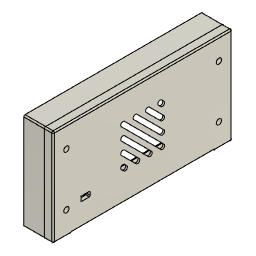
matrix (Autodesk Fusion 360 design; units mm, degrees)
Autodesk Fusion 360 part; units mm, degrees
sketch "Sketch1" plane through (0, 0, 0) normal (1, 0, 0) x (0, 1, 0) in component "Matrix"
  line L0 (96, -48) -> (-96, -48)
  line L1 (-96, -48) -> (-96, 48)
  line L2 (-96, 48) -> (96, 48)
  line L3 (96, 48) -> (96, -48)
  line L4 (96, -48) -> (-96, 48) construction
  line L5 (-96, -48) -> (96, 48) construction
  line L6 (-96, 30) -> (96, 30) construction
  line L7 (-96, -30) -> (96, -30) construction
  line L8 (-87, 48) -> (-87, -48) construction
  line L9 (87, 48) -> (87, -48) construction
  line L10 (0, 30) -> (0, -30) construction
  line L11 (-87, 0) -> (87, 0) construction
  circle A0 centre (-87, 30) radius 1.5
  circle A1 centre (-87, -30) radius 1.5
  circle A2 centre (87, -30) radius 1.5
  circle A3 centre (87, 30) radius 1.5
  line L12 (-96, 37) -> (96, 37) construction
  line L13 (-96, -37) -> (96, -37) construction
  line L14 (-12, 48) -> (-12, -48) construction
  line L15 (12, 48) -> (12, -48) construction
  circle A4 centre (12, 37) radius 1.5
  circle A5 centre (-12, -37) radius 1.5
  dimension "d3" = 192
  dimension "d4" = 96
  dimension "d5" = 9
  dimension "d6" = 18
  dimension "d7" = 3
  dimension "d9" = 12
  dimension "d10" = 11
  constraint perpendicular L0 L1
  constraint parallel L0 L2
  constraint parallel L1 L3
  constraint horizontal L0
  constraint coincident L4 origin
  constraint coincident L5 origin
  constraint coincident L1 L6.start
  constraint coincident L3 L6.end
  constraint perpendicular L3 L6
  constraint coincident L1 L7.start
  constraint coincident L3 L7.end
  constraint perpendicular L3 L7
  constraint coincident L2 L8.start
  constraint coincident L0 L8.end
  constraint perpendicular L0 L8
  constraint coincident L2 L9.start
  constraint coincident L0 L9.end
  constraint perpendicular L0 L9
  constraint perpendicular L6 L10
  constraint perpendicular L10 L11
  constraint symmetric L6 L7 L11
  constraint midpoint origin L11
  constraint midpoint origin L10
  constraint midpoint L6 L10.start
  constraint coincident L8 L11.start
  constraint coincident L8 A0.centre
  constraint coincident L6 A0.centre
  constraint coincident L7 A1.centre
  constraint coincident L8 A1.centre
  constraint coincident L9 A2.centre
  constraint coincident L7 A2.centre
  constraint coincident L6 A3.centre
  constraint coincident L9 A3.centre
  constraint equal A2 A3
  constraint equal A0 A3
  constraint equal A0 A1
  constraint coincident L1 L12.start
  constraint coincident L3 L12.end
  constraint perpendicular L3 L12
  constraint coincident L1 L13.start
  constraint coincident L3 L13.end
  constraint perpendicular L3 L13
  constraint coincident L2 L14.start
  constraint coincident L0 L14.end
  constraint perpendicular L0 L14
  constraint coincident L2 L15.start
  constraint coincident L0 L15.end
  constraint perpendicular L0 L15
  constraint symmetric L11 L12 L13
  constraint coincident L12 A4.centre
  constraint coincident L15 A4.centre
  constraint coincident L13 A5.centre
  constraint coincident L14 A5.centre
  constraint equal A4 A5
  constraint equal A0 A5
  measures "d3" distance of L1.end L2.end
  measures "d4" distance of L0.start L2.end
  measures "d5" distance of L1 L8
  measures "d6" distance of L0 L7
  measures "d7" diameter of A0
  measures "d9" distance of L10 L15
  measures "d10" distance of L2 L12
sketch "Sketch3" plane through (0, 0, 0) normal (1, 0, 0) x (0, 1, 0) in component "Matrix"
  line L0 (96, -48) -> (-96, -48)
  line L1 (-96, -48) -> (-96, 48)
  line L2 (96, 48) -> (96, -48)
  line L3 (-96, 48) -> (96, 48)
  circle A0 centre (-87, 30) radius 1.5
  circle A1 centre (-87, -30) radius 1.5
  circle A2 centre (87, -30) radius 1.5
  circle A3 centre (87, 30) radius 1.5
  line L4 (0, 30) -> (0, -30) construction
  line L5 (-87, 0) -> (87, 0) construction
  line L6 (82.25, -35.25) -> (-82.25, -35.25)
  line L7 (-82.25, -35.25) -> (-82.25, 35.25)
  line L8 (-82.25, 35.25) -> (82.25, 35.25)
  line L9 (82.25, 35.25) -> (82.25, -35.25)
  line L10 (82.25, -35.25) -> (-82.25, 35.25) construction
  line L11 (-82.25, -35.25) -> (82.25, 35.25) construction
  circle A4 centre (12, 37) radius 1.5
  circle A5 centre (-12, -37) radius 1.5
  circle A6 centre (-12, -37) radius 4
  circle A7 centre (12, 37) radius 4
  point P0 (-87, -30)
  dimension "d15" = 12.75
  dimension "d16" = 13.75
  dimension "d18" = 8
  constraint perpendicular L6 L7
  constraint parallel L6 L8
  constraint parallel L7 L9
  constraint horizontal L6
  constraint coincident L10 origin
  constraint coincident L11 origin
  constraint concentric A5 A6
  constraint concentric A4 A7
  constraint equal A6 A7
  measures "d15" distance of L3 L8
  measures "d16" distance of L2 L9
  measures "d18" diameter of A6
extrude "Extrude3" add sketch "Sketch3" along normal mid plane 15 contours L0 L1 L2 L3 | A0 | A1 | A2 | A3 | L6 L7 L8 L9 A6 A7 | L6 A6 | L6 A6 | L8 A7 | L8 A7 | A4 | A5 makes body 1 in component "Matrix"
extrude "Extrude4" cut sketch "Sketch3" against normal blind 13 from surface at 7.5 contours L6 L7 L8 L9 A6 A7 bodies 1 in component "Matrix"
extrude "Extrude5" cut sketch "Sketch3" against normal blind 5 from surface at 7.5 contours A0 | A1 | A2 | A3 | A4 | A5 bodies 1 in component "Matrix"
sketch "Sketch1 (2)" plane through (7.5, 0, 0) normal (1, 0, 0) x (0, 1, 0) in component "Fit Test"
  circle A0 centre (87, -30) radius 1.5 construction
  circle A1 centre (87, 30) radius 1.5 construction
  line L0 (96, -48) -> (96, 48) construction
  circle A2 centre (87, 30) radius 1.875
  circle A3 centre (87, -30) radius 1.875
  line L1 (96.5, -48) -> (96.5, 48)
  circle A4 centre (87, 30) radius 5
  circle A5 centre (87, -30) radius 5
  line L2 (87, 35) -> (98.5, 35)
  line L3 (98.5, 35) -> (98.5, -35)
  line L4 (98.5, -35) -> (87, -35)
  line L5 (87, 30) -> (87, -30)
  dimension "d51" = 3.75
  dimension "d52" = 0.5
  dimension "d53" = 10
  dimension "d54" = 2
  constraint concentric A1 A2
  constraint concentric A0 A3
  constraint equal A2 A3
  constraint concentric A1 A4
  constraint concentric A0 A5
  constraint equal A4 A5
  constraint coincident A4 L2.start
  constraint perpendicular L0 L2
  constraint perpendicular L2 L3
  constraint coincident A5 L4.end
  constraint tangent A5 L4
  constraint horizontal L4
  constraint tangent A4 L2
  constraint coincident A1.centre A2.centre
  constraint coincident A0.centre A3.centre
  measures "d51" diameter of A2
  measures "d53" diameter of A4
  measures "d54" distance of L1 L3
extrude "Extrude1" add sketch "Sketch1 (2)" along normal blind 2 separate body makes body 2 in component "Fit Test"
extrude "Extrude2" add sketch "Sketch1 (2)" against normal blind 3 contours L1 L2 L3 L4 bodies 2 in component "Fit Test"
ref_plane "WorkPlane1" through (-8, 0, 0) normal (-1, 0, 0) x (0, 0, 1) in component "Perspex"
sketch "Sketch1 (3)" plane through (-8, 0, 0) normal (-1, 0, 0) x (0, 1, 0) in component "Perspex"
  line L0 (-99, 51) -> (99, 51)
  line L1 (99, 51) -> (99, -51)
  line L2 (99, -51) -> (-99, -51)
  line L3 (-99, -51) -> (-99, 51)
  line L4 (-99, 51) -> (99, -51) construction
  line L5 (99, 51) -> (-99, -51) construction
  dimension "d28" = 198
  dimension "d29" = 102
  constraint perpendicular L0 L1
  constraint parallel L0 L2
  constraint parallel L1 L3
  constraint horizontal L0
  constraint coincident L4 origin
  constraint coincident L5 origin
  measures "d28" distance of L1.end L2.end
  measures "d29" distance of L0 L2
extrude "Extrude1'" add sketch "Sketch1 (3)" along normal blind 3 separate body makes body 3 in component "Perspex"
sketch "Sketch1 (4)" plane through (-8, 0, 0) normal (1, 0, 0) x (0, 1, 0) in component "Case"
  line L0 (99, 51) -> (-99, 51) construction
  line L1 (-99, 51) -> (-99, -51) construction
  line L2 (-99, -51) -> (99, -51) construction
  line L3 (99, -51) -> (99, 51) construction
  line L4 (96, 48) -> (-96, 48) construction
  line L5 (-96, 48) -> (-96, -48) construction
  line L6 (-96, -48) -> (96, -48) construction
  line L7 (96, -48) -> (96, 48) construction
  line L8 (-96.2, -48.2) -> (96.2, -48.2)
  line L9 (96.2, -48.2) -> (96.2, 48.2)
  line L10 (96.2, 48.2) -> (-96.2, 48.2)
  line L11 (-96.2, 48.2) -> (-96.2, -48.2)
  line L12 (-99.2, -51.2) -> (99.2, -51.2)
  line L13 (99.2, -51.2) -> (99.2, 51.2)
  line L14 (99.2, 51.2) -> (-99.2, 51.2)
  line L15 (-99.2, 51.2) -> (-99.2, -51.2)
  line L16 (102.2, -54.2) -> (-102.2, -54.2)
  line L17 (-102.2, -54.2) -> (-102.2, 54.2)
  line L18 (-102.2, 54.2) -> (102.2, 54.2)
  line L19 (102.2, 54.2) -> (102.2, -54.2)
  line L20 (102.2, -54.2) -> (-102.2, 54.2) construction
  line L21 (-102.2, -54.2) -> (102.2, 54.2) construction
  dimension "d32" = 0.2
  dimension "d33" = 0.2
  dimension "d34" = 3
  dimension "d35" = 3
  constraint perpendicular L16 L17
  constraint parallel L16 L18
  constraint parallel L17 L19
  constraint horizontal L16
  constraint coincident L20 origin
  constraint coincident L21 origin
  measures "d34" distance of L14 L18
  measures "d35" distance of L13 L19
extrude "Extrude1''" add sketch "Sketch1 (4)" against normal up to surface (4 mm away) separate body contours L16 L17 L18 L19 makes body 4 in component "Case"
extrude "Extrude2'" add sketch "Sketch1 (4)" along normal up to surface (15.5 mm away) contours L12 L13 L14 L15 | L16 L17 L18 L19 bodies 4 in component "Case"
sketch "Sketch2" plane through (7.5, 0, 0) normal (1, 0, 0) x (0, 1, 0) in component "Case"
  circle A0 centre (-87, 30) radius 1.5 construction
  circle A1 centre (-87, -30) radius 1.5 construction
  circle A2 centre (87, -30) radius 1.5 construction
  circle A3 centre (87, 30) radius 1.5 construction
  line L0 (96.2, -48.2) -> (-96.2, -48.2)
  line L1 (-96.2, -48.2) -> (-96.2, 48.2)
  line L2 (-96.2, 48.2) -> (96.2, 48.2)
  line L3 (96.2, 48.2) -> (96.2, -48.2)
  line L4 (102.2, -54.2) -> (102.2, 54.2)
  line L5 (102.2, 54.2) -> (-102.2, 54.2)
  line L6 (-102.2, 54.2) -> (-102.2, -54.2)
  line L7 (-102.2, -54.2) -> (102.2, -54.2)
  line L8 (-87, 34.25) -> (-96.2, 34.25)
  line L9 (-87, 25.75) -> (-96.2, 25.75)
  line L10 (-87, -25.75) -> (-96.2, -25.75)
  line L11 (-87, -34.25) -> (-96.2, -34.25)
  line L12 (87, 34.25) -> (96.2, 34.25)
  line L13 (87, 25.75) -> (96.2, 25.75)
  line L14 (87, -25.75) -> (96.2, -25.75)
  line L15 (87, -34.25) -> (96.2, -34.25)
  arc A4 (-87, 25.75) -> (-87, 34.25) centre (-87, 30) ccw
  arc A5 (-87, -34.25) -> (-87, -25.75) centre (-87, -30) ccw
  arc A6 (87, -25.75) -> (87, -34.25) centre (87, -30) ccw
  arc A7 (87, 34.25) -> (87, 25.75) centre (87, 30) ccw
  circle A8 centre (-87, 30) radius 1.75
  circle A9 centre (-87, -30) radius 1.75
  circle A10 centre (87, -30) radius 1.75
  circle A11 centre (87, 30) radius 1.75
  dimension "d42" = 3.5
  dimension "d289" = 2.5
  constraint concentric A0 A4
  constraint concentric A1 A5
  constraint concentric A2 A6
  constraint concentric A3 A7
  constraint equal A6 A7
  constraint equal A4 A7
  constraint equal A4 A5
  constraint coincident L1 L8.end
  constraint tangent L8 A4
  constraint coincident L1 L9.end
  constraint tangent L9 A4
  constraint coincident L1 L10.end
  constraint tangent L10 A5
  constraint coincident L1 L11.end
  constraint tangent L11 A5
  constraint coincident L3 L12.end
  constraint tangent L12 A7
  constraint coincident L3 L13.end
  constraint tangent L13 A7
  constraint coincident L3 L14.end
  constraint tangent L14 A6
  constraint coincident L3 L15.end
  constraint tangent L15 A6
  constraint parallel L13 L15
  constraint perpendicular L3 L12
  constraint perpendicular L3 L13
  constraint perpendicular L3 L14
  constraint perpendicular L1 L8
  constraint perpendicular L1 L9
  constraint perpendicular L1 L10
  constraint perpendicular L1 L11
  constraint concentric A0 A8
  constraint concentric A1 A9
  constraint concentric A2 A10
  constraint concentric A7 A11
  constraint equal A8 A9
  constraint equal A8 A11
  constraint equal A10 A11
  measures "d42" diameter of A8
  measures "d289" distance of A4 A8
extrude "Extrude3'" add sketch "Sketch2" along normal blind 4 contours L3 L14 L15 A6 | L1 L10 L11 A5 | L3 L12 L13 A7 | L1 L8 L9 A4 | L4 L5 L6 L7 bodies 4 in component "Case"
ref_plane "WorkPlane1" through (7.5, 0, 0) normal (1, 0, 0) x (0, 0, -1) in component "Case"
sketch "Sketch4" plane through (7.5, 0, 0) normal (1, 0, 0) x (0, 1, 0) in component "Case"
  line L0 (-96, 48) -> (-96, -48) construction
  line L1 (96.2, -48.2) -> (-96.2, -48.2)
  circle A0 centre (-18.5, -29) radius 1.75
  line L2 (-96.2, 48.2) -> (96.2, 48.2)
  line L3 (-21.7368, -28.7072) -> (-23.5, -48.2)
  line L4 (-15.2632, -28.7072) -> (-13.5, -48.2)
  arc A1 (-15.2632, -28.7072) -> (-21.7368, -28.7072) centre (-18.5, -29) ccw
  line L5 (30.5, 29) -> (-18.5, -29) construction
  line L6 (6, 0) -> (6, 48.2) construction
  line L7 (-18.5, -29) -> (-18.5, -48.2) construction
  line L8 (6, 0) -> (-75.1165, 0) construction
  dimension "d69" = 49
  dimension "d73" = 58
  dimension "d190" = 3.5
  dimension "d194" = 10
  dimension "d291" = 1.5
  dimension "d322" = 6
  constraint concentric A0 A1
  constraint coincident L1 L3.end
  constraint tangent L3 A1
  constraint coincident L1 L4.end
  constraint tangent L4 A1
  constraint vertical L6
  constraint coincident A0.centre A1.centre
  constraint coincident L1 L7.end
  constraint perpendicular L1 L7
  constraint symmetric L3 L4 L7
  constraint horizontal L8
  constraint coincident L5 L6.start
  constraint coincident origin L8
  constraint coincident L2 L6.end
  constraint midpoint L5 L6.start
  measures "d69" horizontal distance of A0.centre L5.start
  measures "d73" vertical distance of A0.centre L5.start
  measures "d190" diameter of A0
  measures "d194" distance of L3.end L4.end
  measures "d291" distance of A0 A1
  measures "d322" distance of origin L6.start
extrude "Extrude5'" add sketch "Sketch4" along normal up to surface (4 mm away) bodies 4 in component "Case"
mirror "Mirror3" about plane through (0, 0, 0) normal (0, 0, 1) of "Extrude5'" in component "Case"
ref_plane "WorkPlane2" through (7.5, 6, 0) normal (0, -1, 0) x (1, 0, 0) in component "Case"
mirror "Mirror4" about plane through (7.5, 6, 0) normal (0, -1, 0) of "Extrude5'", "Mirror3" in component "Case"
sketch "Sketch7" plane through (11.5, 0, 0) normal (1, 0, 0) x (0, 1, 0) in component "Case"
  line L0 (-96.2, 48.2) -> (-23.5, 48.2)
  line L1 (96.2, 48.2) -> (96.2, 34.25)
  line L2 (96.2, 34.25) -> (87, 34.25)
  arc A0 (87, 34.25) -> (87, 25.75) centre (87, 30) ccw
  line L3 (87, 25.75) -> (96.2, 25.75)
  line L4 (96.2, -25.75) -> (87, -25.75)
  arc A1 (87, -25.75) -> (87, -34.25) centre (87, -30) ccw
  line L5 (87, -34.25) -> (96.2, -34.25)
  line L6 (96.2, -48.2) -> (35.5, -48.2)
  line L7 (-96.2, 34.25) -> (-96.2, 48.2)
  line L8 (-96.2, -34.25) -> (-87, -34.25)
  arc A2 (-87, -34.25) -> (-87, -25.75) centre (-87, -30) ccw
  line L9 (-87, -25.75) -> (-96.2, -25.75)
  line L10 (-96.2, 25.75) -> (-87, 25.75)
  arc A3 (-87, 25.75) -> (-87, 34.25) centre (-87, 30) ccw
  line L11 (-87, 34.25) -> (-96.2, 34.25)
  circle A4 centre (-87, -30) radius 1.75
  circle A5 centre (87, 30) radius 1.75
  circle A6 centre (87, -30) radius 1.75
  circle A7 centre (-87, 30) radius 1.75
  line L12 (-102.2, -54.2) -> (102.2, -54.2)
  line L13 (102.2, -54.2) -> (102.2, 54.2)
  line L14 (102.2, 54.2) -> (-102.2, 54.2)
  line L15 (-102.2, 54.2) -> (-102.2, -54.2)
  line L16 (17.694, -48.2) -> (35.5, -48.2)
  line L17 (35.5, -48.2) -> (35.5, -17.1281)
  line L18 (35.5, -17.1281) -> (17.694, -17.1281)
  line L19 (17.694, -17.1281) -> (17.694, -48.2)
  line L20 (-29.5, 48.2) -> (-8.6042, 48.2)
  line L21 (-8.6042, 48.2) -> (-8.6042, 21.8764)
  line L22 (-8.6042, 21.8764) -> (-29.5, 21.8764)
  line L23 (-29.5, 21.8764) -> (-29.5, 48.2)
  circle A8 centre (30.5, 29) radius 1.75
  circle A9 centre (-18.5, 29) radius 1.75
  circle A10 centre (-18.5, -29) radius 1.75
  line L24 (-23.5, 48.2) -> (-21.7368, 28.7072)
  arc A11 (-21.7368, 28.7072) -> (-15.2632, 28.7072) centre (-18.5, 29) ccw
  line L25 (-15.2632, 28.7072) -> (-13.5, 48.2)
  line L26 (-13.5, 48.2) -> (25.5, 48.2)
  line L27 (25.5, 48.2) -> (27.2632, 28.7072)
  arc A12 (27.2632, 28.7072) -> (33.7368, 28.7072) centre (30.5, 29) ccw
  line L28 (33.7368, 28.7072) -> (35.5, 48.2)
  line L29 (96.2, 25.75) -> (96.2, -25.75)
  line L30 (96.2, -34.25) -> (96.2, -48.2)
  line L31 (-13.5, -48.2) -> (-15.2632, -28.7072)
  arc A13 (-15.2632, -28.7072) -> (-21.7368, -28.7072) centre (-18.5, -29) ccw
  line L32 (-21.7368, -28.7072) -> (-23.5, -48.2)
  line L33 (-23.5, -48.2) -> (-96.2, -48.2)
  line L34 (-96.2, -25.75) -> (-96.2, 25.75)
  circle A14 centre (30.5, -29) radius 1.75
  line L35 (35.5, 48.2) -> (96.2, 48.2)
  line L36 (35.5, -48.2) -> (33.7368, -28.7072)
  arc A15 (33.7368, -28.7072) -> (27.2632, -28.7072) centre (30.5, -29) ccw
  line L37 (27.2632, -28.7072) -> (25.5, -48.2)
  line L38 (25.5, -48.2) -> (-13.5, -48.2)
  line L39 (-96.2, -48.2) -> (-96.2, -34.25)
  constraint horizontal L16
  constraint vertical L17
  constraint horizontal L18
  constraint vertical L19
  constraint coincident L6.end L17
  constraint horizontal L20
  constraint vertical L21
  constraint horizontal L22
  constraint vertical L23
extrude "Extrude13" cut sketch "Sketch7" against normal blind 13 contours L0 L20 L21 L22 L23 L24 A11 L25 L26 | L20 L24 A11 L25 | L16 L17 L18 L19 L36 A15 L37 L38 | L16 L36 A15 L37 | A9 | A14 bodies 4 in component "Case"
sketch "Sketch11" plane through (0, 0, -54.2) normal (0, 0, -1) x (1, 0, 0) in component "Case"
  line L0 (-12, 102.2) -> (-12, -102.2)
  line L1 (-12, -102.2) -> (11.5, -102.2)
  line L2 (11.5, -102.2) -> (11.5, 102.2)
  line L3 (11.5, 102.2) -> (-12, 102.2)
  line L4 (-12, 82.2) -> (11.5, 82.2)
  dimension "d295" = 20
  constraint coincident L0 L4.start
  constraint coincident L2 L4.end
  constraint perpendicular L2 L4
  measures "d295" distance of L3 L4
extrude "Extrude16" add sketch "Sketch11" along normal blind 2 contours L0 L2 L3 L4 bodies 4 in component "Case"
mirror "Mirror5" about plane through (0, 0, 0) normal (0, 1, 0) of "Extrude16" in component "Case"
fillet "Fillet7" radius 1 2 edges at (-0.25, -82.2, -54.2) (-0.25, 82.2, -54.2) on bodies 4 in component "Case"
sketch "Sketch1 (5)" plane through (11.5, 0, 0) normal (1, 0, 0) x (0, 1, 0) in component "Back"
  line L0 (-81.2, -54.2) -> (81.2, -54.2)
  arc A0 (82.2, -55.2) -> (81.2, -54.2) centre (81.2, -55.2) ccw
  line L1 (82.2, -55.2) -> (82.2, -56.2)
  line L2 (82.2, -56.2) -> (102.2, -56.2)
  line L3 (102.2, -56.2) -> (102.2, 54.2)
  line L4 (102.2, 54.2) -> (-102.2, 54.2)
  line L5 (-102.2, 54.2) -> (-102.2, -56.2)
  line L6 (-102.2, -56.2) -> (-82.2, -56.2)
  line L7 (-82.2, -56.2) -> (-82.2, -55.2)
  arc A1 (-81.2, -54.2) -> (-82.2, -55.2) centre (-81.2, -55.2) ccw
  circle A2 centre (87, -30) radius 1.75
  circle A3 centre (87, 30) radius 1.75
  circle A4 centre (-87, 30) radius 1.75
  line L8 (96.2, -48.2) -> (-13.5, -48.2)
  line L9 (-96.2, -48.2) -> (-96.2, -34.25)
  line L10 (-96.2, 25.75) -> (-87, 25.75)
  arc A5 (-87, 25.75) -> (-87, 34.25) centre (-87, 30) ccw
  line L11 (-87, 34.25) -> (-96.2, 34.25)
  line L12 (-96.2, 48.2) -> (25.5, 48.2)
  line L13 (96.2, 48.2) -> (96.2, 34.25)
  line L14 (96.2, 34.25) -> (87, 34.25)
  arc A6 (87, 34.25) -> (87, 25.75) centre (87, 30) ccw
  line L15 (87, 25.75) -> (96.2, 25.75)
  line L16 (96.2, -25.75) -> (87, -25.75)
  arc A7 (87, -25.75) -> (87, -34.25) centre (87, -30) ccw
  line L17 (87, -34.25) -> (96.2, -34.25)
  line L18 (25.5, 48.2) -> (35.5, 48.2)
  line L19 (-29.5, -48.2) -> (-13.5, -48.2)
  line L20 (-13.5, -48.2) -> (-15.2632, -28.7072)
  arc A8 (-15.2632, -28.7072) -> (-21.7368, -28.7072) centre (-18.5, -29) ccw
  line L21 (-21.7368, -28.7072) -> (-23.5, -48.2)
  line L22 (-23.5, -48.2) -> (-96.2, -48.2)
  line L23 (-96.2, -34.25) -> (-87, -34.25)
  arc A9 (-87, -34.25) -> (-87, -25.75) centre (-87, -30) ccw
  line L24 (-87, -25.75) -> (-96.2, -25.75)
  line L25 (-96.2, -25.75) -> (-96.2, 25.75)
  line L26 (-96.2, 34.25) -> (-96.2, 48.2)
  line L27 (25.5, 48.2) -> (27.2632, 28.7072)
  arc A10 (27.2632, 28.7072) -> (33.7368, 28.7072) centre (30.5, 29) ccw
  line L28 (33.7368, 28.7072) -> (35.5, 48.2)
  line L29 (35.5, 48.2) -> (96.2, 48.2)
  line L30 (96.2, 25.75) -> (96.2, -25.75)
  line L31 (96.2, -34.25) -> (96.2, -48.2)
  circle A11 centre (30.5, 29) radius 1.75
  circle A12 centre (-18.5, -29) radius 1.75
  circle A13 centre (-87, -30) radius 1.75
  constraint coincident L12.end L18.start
  constraint coincident L8.end L19.end
  constraint coincident L18.end L28.end
extrude "Extrude1'''" add sketch "Sketch1 (5)" along normal blind 8 separate body contours L0 A0 L1 L2 L3 L4 L5 L6 L7 A1 makes body 5 in component "Back"
sketch "Sketch13" plane through (19.5, 0, 0) normal (1, 0, 0) x (0, 1, 0) in component "Back"
  circle A0 centre (87, -30) radius 1.75
  line L0 (96.2, -48.2) -> (-96.2, -48.2) construction
  line L1 (-96.2, -48.2) -> (-96.2, -34.25) construction
  line L2 (-96.2, 25.75) -> (-87, 25.75) construction
  arc A1 (-87, 25.75) -> (-87, 34.25) centre (-87, 30) ccw construction
  line L3 (-87, 34.25) -> (-96.2, 34.25) construction
  line L4 (-96.2, 48.2) -> (96.2, 48.2) construction
  line L5 (96.2, 48.2) -> (96.2, 34.25) construction
  line L6 (96.2, 34.25) -> (87, 34.25) construction
  arc A2 (87, 34.25) -> (87, 25.75) centre (87, 30) ccw construction
  line L7 (87, 25.75) -> (96.2, 25.75) construction
  line L8 (96.2, -25.75) -> (87, -25.75) construction
  arc A3 (87, -25.75) -> (87, -34.25) centre (87, -30) ccw construction
  line L9 (87, -34.25) -> (96.2, -34.25) construction
  circle A4 centre (-87, 30) radius 1.75
  circle A5 centre (87, 30) radius 1.75
  line L10 (82.2, -55.2) -> (82.2, -56.2)
  line L11 (82.2, -56.2) -> (102.2, -56.2)
  line L12 (102.2, -56.2) -> (102.2, 54.2)
  line L13 (102.2, 54.2) -> (-102.2, 54.2)
  line L14 (-102.2, 54.2) -> (-102.2, -56.2)
  line L15 (-102.2, -56.2) -> (-82.2, -56.2)
  line L16 (-82.2, -56.2) -> (-82.2, -55.2)
  arc A6 (-81.2, -54.2) -> (-82.2, -55.2) centre (-81.2, -55.2) ccw
  line L17 (-81.2, -54.2) -> (81.2, -54.2)
  arc A7 (82.2, -55.2) -> (81.2, -54.2) centre (81.2, -55.2) ccw
  line L18 (-96.2, -34.25) -> (-87, -34.25)
  arc A8 (-87, -34.25) -> (-87, -25.75) centre (-87, -30) ccw
  line L19 (-87, -25.75) -> (-96.2, -25.75)
  line L20 (-96.2, -25.75) -> (-96.2, 25.75)
  line L21 (-96.2, 34.25) -> (-96.2, 48.2)
  line L22 (96.2, 25.75) -> (96.2, -25.75)
  line L23 (96.2, -34.25) -> (96.2, -48.2)
  circle A9 centre (-87, -30) radius 1.75
  line L24 (96.2, 48.2) -> (106.2, 48.2)
  constraint coincident L4.end L5.start
extrude "Extrude12" add sketch "Sketch13" along normal blind 2 bodies 5 in component "Back"
sketch "Sketch15" plane through (21.5, 0, 0) normal (1, 0, 0) x (0, 1, 0) in component "Back"
  circle A0 centre (87, -30) radius 1.75
  circle A1 centre (-87, 30) radius 1.75
  circle A2 centre (87, 30) radius 1.75
  line L0 (82.2, -56.2) -> (102.2, -56.2)
  line L1 (102.2, -56.2) -> (102.2, 54.2)
  line L2 (102.2, 54.2) -> (-102.2, 54.2)
  line L3 (-102.2, 54.2) -> (-102.2, -56.2)
  line L4 (-102.2, -56.2) -> (-82.2, -56.2)
  line L5 (-82.2, -56.2) -> (-82.2, -55.2)
  arc A3 (-81.2, -54.2) -> (-82.2, -55.2) centre (-81.2, -55.2) ccw
  line L6 (-81.2, -54.2) -> (81.2, -54.2)
  arc A4 (82.2, -55.2) -> (81.2, -54.2) centre (81.2, -55.2) ccw
  line L7 (82.2, -55.2) -> (82.2, -56.2)
  circle A5 centre (-87, 30) radius 1.75
  circle A6 centre (87, 30) radius 1.75
  circle A7 centre (87, -30) radius 1.75
  circle A8 centre (-87, 30) radius 3
  circle A9 centre (-87, -30) radius 3
  circle A10 centre (87, -30) radius 3
  circle A11 centre (87, 30) radius 3
  circle A12 centre (-87, -30) radius 1.75
  circle A13 centre (-87, -30) radius 1.75
  dimension "d316" = 6
  constraint coincident A1.centre A5.centre
  constraint concentric A7 A10
  constraint concentric A2 A11
  constraint equal A8 A9
  constraint equal A9 A10
  constraint equal A10 A11
  constraint coincident A9.centre A12.centre
  measures "d316" diameter of A8
extrude "Extrude14" cut sketch "Sketch15" against normal up to surface (8 mm away) contours A8 | A9 | A10 | A11 bodies 5 in component "Back"
sketch "Sketch6" plane through (19.5, 0, 0) normal (-1, 0, 0) x (0, -1, 0) in component "Back"
  line L0 (70.25, -30.25) -> (59.85, -30.25)
  line L1 (59.85, -30.25) -> (59.85, -24.85)
  line L2 (59.85, -24.85) -> (70.25, -24.85)
  line L3 (70.25, -24.85) -> (70.25, -30.25)
  line L4 (70.25, -30.25) -> (59.85, -24.85) construction
  line L5 (59.85, -30.25) -> (70.25, -24.85) construction
  line L6 (-96.2, -48.2) -> (96.2, -48.2)
  line L7 (96.2, -48.2) -> (96.2, -34.25)
  line L8 (96.2, 25.75) -> (87, 25.75)
  arc A0 (87, 34.25) -> (87, 25.75) centre (87, 30) ccw
  line L9 (87, 34.25) -> (96.2, 34.25)
  line L10 (96.2, 48.2) -> (-96.2, 48.2)
  line L11 (-96.2, 48.2) -> (-96.2, 34.25)
  line L12 (-96.2, 34.25) -> (-87, 34.25)
  arc A1 (-87, 25.75) -> (-87, 34.25) centre (-87, 30) ccw
  line L13 (-87, 25.75) -> (-96.2, 25.75)
  line L14 (-96.2, -25.75) -> (-87, -25.75)
  arc A2 (-87, -34.25) -> (-87, -25.75) centre (-87, -30) ccw
  line L15 (-87, -34.25) -> (-96.2, -34.25)
  line L16 (-82.25, -35.25) -> (8.4031, -35.25)
  line L17 (-82.25, 35.25) -> (-82.25, -35.25)
  line L18 (-96.2, -34.25) -> (-96.2, -48.2)
  line L19 (96.2, -34.25) -> (87, -34.25)
  arc A3 (87, -25.75) -> (87, -34.25) centre (87, -30) ccw
  line L20 (87, -25.75) -> (96.2, -25.75)
  line L21 (96.2, -25.75) -> (96.2, 25.75)
  line L22 (96.2, 34.25) -> (96.2, 48.2)
  line L23 (-96.2, 25.75) -> (-96.2, -25.75)
  line L24 (82.25, -35.25) -> (82.25, 35.25)
  point P0 (65.05, -27.55)
  dimension "d150" = 10.4
  dimension "d151" = 5.4
  dimension "d303" = 5
  dimension "d326" = 12
  constraint perpendicular L0 L1
  constraint parallel L0 L2
  constraint parallel L1 L3
  constraint horizontal L0
  constraint coincident L4 P0
  constraint coincident L5 P0
  measures "d150" distance of L1.end L2.end
  measures "d151" distance of L0.start L2.end
  measures "d303" distance of L0 L16
  measures "d326" distance of L3 L24
extrude "Extrude7" cut sketch "Sketch6" against normal blind 13 contours L0 L1 L2 L3 bodies 5 in component "Back"
chamfer "Chamfer1" distance 1 angle 45 2 edges at (20.5, -59.85, -24.85) (20.5, -59.85, -30.25) on bodies 5 in component "Back"
sketch "Sketch16" plane through (19.5, 0, 0) normal (-1, 0, 0) x (0, -1, 0) in component "Back"
  line L0 (59.85, -29.25) -> (59.85, -25.85)
  line L1 (59.85, -25.85) -> (60.85, -24.85)
  line L2 (60.85, -24.85) -> (70.25, -24.85)
  line L3 (70.25, -24.85) -> (70.25, -30.25)
  line L4 (70.25, -30.25) -> (60.85, -30.25)
  line L5 (60.85, -30.25) -> (59.85, -29.25)
  line L6 (-96.2, -34.25) -> (-96.2, -48.2)
  line L7 (-96.2, -48.2) -> (96.2, -48.2)
  line L8 (96.2, -48.2) -> (96.2, -34.25)
  line L9 (96.2, -34.25) -> (87, -34.25)
  arc A0 (87, -25.75) -> (87, -34.25) centre (87, -30) ccw
  line L10 (87, -25.75) -> (96.2, -25.75)
  line L11 (96.2, -25.75) -> (96.2, 25.75)
  line L12 (96.2, 25.75) -> (87, 25.75)
  arc A1 (87, 34.25) -> (87, 25.75) centre (87, 30) ccw
  line L13 (87, 34.25) -> (96.2, 34.25)
  line L14 (96.2, 34.25) -> (96.2, 48.2)
  line L15 (96.2, 48.2) -> (-96.2, 48.2)
  line L16 (-96.2, 48.2) -> (-96.2, 34.25)
  line L17 (-96.2, 34.25) -> (-87, 34.25)
  arc A2 (-87, 25.75) -> (-87, 34.25) centre (-87, 30) ccw
  line L18 (-87, 25.75) -> (-96.2, 25.75)
  line L19 (-96.2, 25.75) -> (-96.2, -25.75)
  line L20 (-96.2, -25.75) -> (-87, -25.75)
  arc A3 (-87, -34.25) -> (-87, -25.75) centre (-87, -30) ccw
  line L21 (-87, -34.25) -> (-96.2, -34.25)
  line L22 (72.25, -32.25) -> (60.0216, -32.25)
  line L23 (60.0216, -32.25) -> (57.85, -30.0784)
  line L24 (57.85, -30.0784) -> (57.85, -25.0216)
  line L25 (57.85, -25.0216) -> (60.0216, -22.85)
  line L26 (60.0216, -22.85) -> (72.25, -22.85)
  line L27 (72.25, -22.85) -> (72.25, -32.25)
  dimension "d323" = -2
extrude "Extrude15" add sketch "Sketch16" along normal blind 2 contours L22 L23 L24 L25 L26 L27 bodies 5 in component "Back"
sketch "Sketch14" plane through (19.5, 0, 0) normal (-1, 0, 0) x (0, -1, 0) in component "Back"
  line L0 (-96.2, -48.2) -> (96.2, -48.2)
  line L1 (96.2, -48.2) -> (96.2, -34.25)
  line L2 (96.2, 25.75) -> (87, 25.75)
  arc A0 (87, 34.25) -> (87, 25.75) centre (87, 30) ccw
  line L3 (87, 34.25) -> (96.2, 34.25)
  line L4 (96.2, 48.2) -> (-96.2, 48.2)
  line L5 (-96.2, 48.2) -> (-96.2, 34.25)
  line L6 (-96.2, 34.25) -> (-87, 34.25)
  arc A1 (-87, 25.75) -> (-87, 34.25) centre (-87, 30) ccw
  line L7 (-87, 25.75) -> (-96.2, 25.75)
  line L8 (-96.2, -25.75) -> (-87, -25.75)
  arc A2 (-87, -34.25) -> (-87, -25.75) centre (-87, -30) ccw
  line L9 (-87, -34.25) -> (-96.2, -34.25)
  line L10 (0, 48.2) -> (0, -48.2) construction
  line L11 (25, -25) -> (-25, -25)
  line L12 (-25, -25) -> (-25, 25)
  line L13 (-25, 25) -> (25, 25)
  line L14 (25, 25) -> (25, -25)
  line L15 (25, -25) -> (-25, 25) construction
  line L16 (-25, -25) -> (25, 25) construction
  line L17 (-28.5355, -25) -> (21.4645, 25)
  line L18 (-49.7487, -3.7868) -> (0.2513, 46.2132)
  line L19 (-46.2132, -7.3223) -> (3.7868, 42.6777)
  line L20 (-42.6777, -10.8579) -> (7.3223, 39.1421)
  line L21 (-39.1421, -14.3934) -> (10.8579, 35.6066)
  line L22 (-35.6066, -17.9289) -> (14.3934, 32.0711)
  line L23 (-32.0711, -21.4645) -> (17.9289, 28.5355)
  line L24 (-25, -28.5355) -> (25, 21.4645)
  line L25 (-21.4645, -32.0711) -> (28.5355, 17.9289)
  line L26 (-17.9289, -35.6066) -> (32.0711, 14.3934)
  line L27 (-14.3934, -39.1421) -> (35.6066, 10.8579)
  line L28 (-10.8579, -42.6777) -> (39.1421, 7.3223)
  line L29 (-7.3223, -46.2132) -> (42.6777, 3.7868)
  line L30 (-3.7868, -49.7487) -> (46.2132, 0.2513)
  line L31 (-96.2, -34.25) -> (-96.2, -48.2)
  line L32 (96.2, -34.25) -> (87, -34.25)
  arc A3 (87, -25.75) -> (87, -34.25) centre (87, -30) ccw
  line L33 (87, -25.75) -> (96.2, -25.75)
  line L34 (96.2, -25.75) -> (96.2, 25.75)
  line L35 (96.2, 34.25) -> (96.2, 48.2)
  line L36 (-96.2, 25.75) -> (-96.2, -25.75)
  line L37 (72.25, -22.85) -> (72.25, -32.25)
  line L38 (72.25, -32.25) -> (60.0216, -32.25)
  line L39 (60.0216, -32.25) -> (57.85, -30.0784)
  line L40 (57.85, -30.0784) -> (57.85, -25.0216)
  line L41 (57.85, -25.0216) -> (60.0216, -22.85)
  line L42 (60.0216, -22.85) -> (72.25, -22.85)
  dimension "d304" = 50
  dimension "d305" = 50
  dimension "d306" = 2.5
  dimension "d309" = -5
  dimension "d310" = 0
  constraint midpoint L4 L10.start
  constraint midpoint L0 L10.end
  constraint horizontal L11
  constraint perpendicular L11 L12
  constraint parallel L11 L13
  constraint parallel L12 L14
  constraint coincident L15 origin
  constraint coincident L16 origin
  constraint coincident L13 L17.end
  constraint horizontal L11.end L17.start
  constraint parallel L16 L17
  measures "d304" distance of L12.end L13.end
  measures "d305" distance of L11 L13
  measures "d306" distance of origin L17
extrude "Extrude13'" cut sketch "Sketch14" against normal blind 8 contours L11 L14 L29 L30 | L11 L14 L27 L28 | L11 L14 L25 L26 | L11 L12 L13 L14 L17 L24 | L12 L13 L22 L23 | L12 L13 L20 L21 | L12 L13 L18 L19 bodies 5 in component "Back"
fillet "Fillet5" radius 2.5 30 edges at (20.5, -25, 21.4645) (20.5, -25, 25) (20.5, -21.4645, 25) (20.5, 25, -21.4645) (20.5, 25, -25) (20.5, 21.4645, -25) (20.5, 25, -14.3934) (20.5, 25, -7.3223) (20.5, 7.3223, -25) (20.5, 14.3934, -25) (20.5, 0.2513, -25) (20.5, -13.8909, -25) (20.5, 25, 6.8198) (20.5, 25, 20.9619) (20.5, 25, -0.2513) (20.5, -6.8198, -25) (20.5, -25, 7.3223) (20.5, -25, -6.8198) (20.5, -25, -20.9619) (20.5, -20.9619, -25) (20.5, -7.3223, 25) (20.5, 6.8198, 25) (20.5, 20.9619, 25) (20.5, -14.3934, 25) (20.5, -0.2513, 25) (20.5, 13.8909, 25) (20.5, 25, 13.8909) (20.5, -25, -13.8909) (20.5, -25, 0.2513) (20.5, -25, 14.3934) on bodies 5 in component "Back"
fillet "Fillet6" radius 1.5 4 edges at (16.5, -102.2, 54.2) (16.5, 102.2, 54.2) (16.5, -102.2, -56.2) (16.5, 102.2, -56.2) on bodies 5 in component "Back"
fillet "Fillet8" radius 1.5 4 edges at (-0.25, -102.2, 54.2) (-0.25, 102.2, 54.2) (-0.25, -102.2, -56.2) (-0.25, 102.2, -56.2) on bodies 4 in component "Case"
fillet "Fillet7'" radius 1.5 9 edges at (21.5, 102.2, -1) (21.5, 0, 54.2) (21.5, 101.7607, 53.7607) (21.5, 91.45, -56.2) (21.5, 101.7607, -55.7607) (21.5, -101.7607, 53.7607) (21.5, -102.2, -1) (21.5, -101.7607, -55.7607) (21.5, -91.45, -56.2) on bodies 5 in component "Back"
component "Matrix" placed x (1, 0, 0) y (0, 1, 0) z (0, 0, 1) at (0, 0, 0)
component "Fit Test" placed x (1, 0, 0) y (0, 1, 0) z (0, 0, 1) at (0, 0, 0)
component "Perspex" placed x (1, 0, 0) y (0, 1, 0) z (0, 0, 1) at (0, 0, 0)
component "Case" placed x (1, 0, 0) y (0, 1, 0) z (0, 0, 1) at (0, 0, 0)
component "Back" placed x (1, 0, 0) y (0, 1, 0) z (0, 0, 1) at (0, 0, 0)
equation "d35 = d34"
equation "d150 = 10.20 mm + 0.2 mm"
equation "d151 = 5.2 mm + 0.2 mm"
